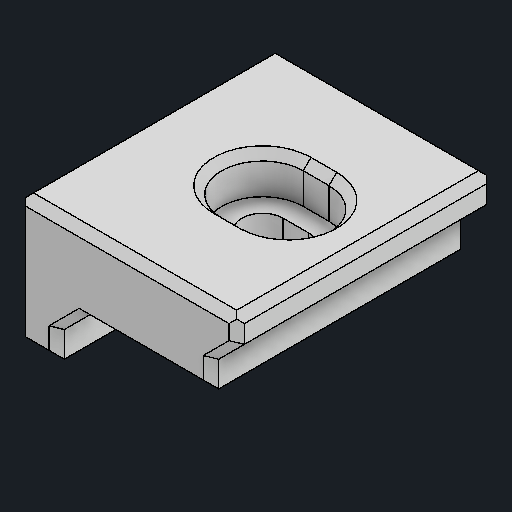
# Autodesk Inventor part: Part1
Saved by Autodesk Inventor 2026.2 (Build 302298000, 298)
## iProperties
Created: 2026-07-19
Part Number: Part1
Material: Generic
Document SubType Name: Modeling
Designer: JoshuaEah
Density: 1 g/cm^3
Appearance: Default
Author: JoshuaEah
Autodesk Inventor part; units mm, degrees
ref_plane "YZ Plane" through (0, 0, 0) normal (1, 0, 0) x (0, 1, 0)
ref_plane "XZ Plane" through (0, 0, 0) normal (0, 1, 0) x (-1, 0, 0)
ref_plane "XY Plane" through (0, 0, 0) normal (0, 0, 1) x (1, 0, 0)
sketch "Sketch1" plane through (0, 0, 0) normal (0, 0, 1) x (1, 0, 0)
  line L0 (0, 0) -> (3, 0)
  line L1 (3, 0) -> (3, 2)
  line L2 (3, 2) -> (5, 4)
  line L3 (5, 4) -> (15, 4)
  line L4 (17, 10) -> (0, 10)
  line L5 (0, 10) -> (0, 0)
  line L6 (15, 4) -> (15, 6)
  line L7 (15, 6) -> (17, 8)
  line L8 (17, 8) -> (17, 10)
  dimension "d0" = 45
  dimension "d2" = 3
  dimension "d4" = 10
  dimension "d6" = 2
  dimension "d7" = 2
  dimension "d8" = 2
  dimension "d25" = 2
  constraints: 18 end point, 3 parallel, 2 perpendicular, 2 vertical, 1 coincident, 1 horizontal
  measures "d0" angle of L2 L1
  measures "d2" distance between parallel lines of L1 L5
  measures "d4" distance of L2.end L3.end
  measures "d6" horizontal distance of L1.end L2.end
  measures "d7" distance of L0.end L1.end
  measures "d8" distance of L3.end L6.end
  measures "d25" distance of L7.end L4.start
extrude "Extrusion1" add sketch "Sketch1" along normal blind 20
sketch "Sketch2" plane through (0, 10, 0) normal (0, 1, 0) x (1, 0, 0)
  line L0 (7.4, -10) -> (12.6, -10) construction
  line L1 (9, -11.6) -> (11, -11.6)
  line L2 (11, -8.4) -> (9, -8.4)
  arc A0 (9, -8.4) -> (9, -11.6) centre (9, -10) ccw
  arc A1 (11, -11.6) -> (11, -8.4) centre (11, -10) ccw
  line L3 (9, -10) -> (11, -10) construction
  line L4 (9, -13.175) -> (11, -13.175)
  line L5 (11, -6.825) -> (9, -6.825)
  arc A2 (9, -6.825) -> (9, -13.175) centre (9, -10) ccw
  arc A3 (11, -13.175) -> (11, -6.825) centre (11, -10) ccw
  line L6 (5, 0) -> (15, 0) construction
  line L7 (15, 0) -> (15, -20) construction
  line L8 (5, -20) -> (15, -20) construction
  line L9 (5, 0) -> (5, -20) construction
  point P0 (10, -10)
  point P1 (7.4, -10)
  point P2 (12.6, -10)
  point P3 (5.825, -10)
  point P4 (10, -20)
  point P5 (5, -10)
  dimension "d11" = 3.2
  dimension "d16" = 6.35
  dimension "d24" = 2
  constraints: 16 end point, 13 point on circle, 8 tangent, 4 centre point, 4 midpoint, 3 point on line, 2 parallel, 1 coincident, 1 horizontal, 1 horizontal alignment, 1 vertical alignment
  measures "d11" diameter of A1
  measures "d16" diameter of A3
  measures "d24" distance of L3.end A0.centre
extrude "Extrusion2" cut sketch "Sketch2" against normal through all contours A0 L2 A1 L1
extrude "Extrusion3" cut sketch "Sketch2" against normal blind 3 contours A0 L2 A1 L1 | A2 L5 A3 L4
chamfer "Chamfer1" distance 0.6 angle 45 25 edges at (8.5, 10, 20) (8.5, 10, 0) (0, 10, 10) (0, 5, 20) (0, 5, 0) (0, 0, 10) (1.5, 0, 20) (1.5, 0, 0) (16, 7, 20) (15, 5, 20) (10, 4, 20) (4, 3, 20) (3, 1, 20) (3, 1, 0) (4, 3, 0) (10, 4, 0) (15, 5, 0) (16, 7, 0) (14.175, 10, 10) (10, 10, 13.175) (5.825, 10, 10) (10, 10, 6.825) (17, 9, 20) (17, 9, 0) (17, 10, 10)
equation "\"d7\" = d6"
equation "\"d8\" = d7"
equation "\"d25\" = d7"
body "Solid1"
